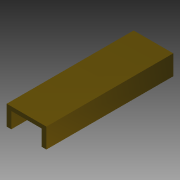
# Autodesk Inventor part: imaginary stopper
Saved by Autodesk Inventor 2011 (Build 150239000, 239)
## iProperties
Created: 2013-01-27
Part Number: imaginary stopper
Document SubType Name: Modeling
Designer: Danny
Density: 1 g/cm^3
Author: Danny
Autodesk Inventor part; units mm, degrees
note: some values were not read from the file. Chosen so that the rebuilt part matches the saved one: second side of "Extrusion1".
ref_plane "YZ Plane" through (0, 0, 0) normal (1, 0, 0) x (0, 1, 0)
ref_plane "XZ Plane" through (0, 0, 0) normal (0, 1, 0) x (-1, 0, 0)
ref_plane "XY Plane" through (0, 0, 0) normal (0, 0, 1) x (1, 0, 0)
sketch "Sketch1" plane through (0, 0, 0) normal (0, 0, 1) x (1, 0, 0)
  line L0 (0, 0) -> (2.921, 0)
  line L1 (25.4, 0) -> (25.4, 12.7)
  line L2 (25.4, 12.7) -> (0, 12.7)
  line L3 (0, 12.7) -> (0, 0)
  line L4 (22.479, 0) -> (22.479, 10.16)
  line L5 (22.479, 10.16) -> (2.921, 10.16)
  line L6 (2.921, 10.16) -> (2.921, 0)
  line L7 (22.479, 0) -> (25.4, 0)
  line L8 (2.921, 0) -> (2.921, 10.16)
  line L9 (22.479, 10.16) -> (22.479, 0)
  constraints: 20 end point, 5 parallel, 2 horizontal, 2 perpendicular, 1 collinear
extrude "Extrusion1" add sketch "Sketch1" along normal blind 76.2
body "Solid1"
